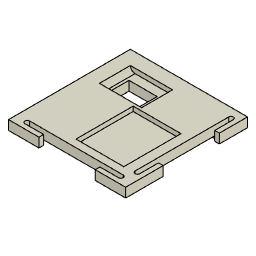
支架2 v23 v1 (Autodesk Fusion 360 design; units mm, degrees)
Autodesk Fusion 360 part; units mm, degrees
sketch "草图1" plane through (0, 0, 0) normal (0, 0, 1) x (1, 0, 0)
  line L0 (57.5, -10) -> (25, -10)
  line L1 (25, -10) -> (25, 0)
  line L2 (25, 0) -> (150, 0)
  line L3 (57.5, -5) -> (57.5, -10)
  line L4 (87.5, 0) -> (117.5, 0)
  arc A0 (137.5, -5) -> (137.5, 0) centre (137.5, -2.5) ccw
  line L5 (150, 30) -> (145, 30)
  arc A1 (37.5, 0) -> (37.5, -5) centre (37.5, -2.5) ccw
  line L6 (150, -10) -> (117.5, -10)
  line L7 (140, 110) -> (140, 60)
  line L8 (150, 120) -> (25, 120)
  line L9 (150, 90) -> (145, 90)
  line L10 (150, 90) -> (150, 120)
  line L11 (87.5, 0) -> (87.5, 120) construction
  line L12 (117.5, -5) -> (117.5, -10)
  line L13 (145, 30) -> (145, 10)
  arc A2 (140, 10) -> (145, 10) centre (142.5, 10) ccw
  line L14 (150, 0) -> (150, 30)
  line L15 (150, 0) -> (150, -10)
  line L16 (137.5, -5) -> (117.5, -5)
  line L17 (140, 10) -> (140, 60)
  line L18 (145, 90) -> (145, 110)
  arc A3 (145, 110) -> (140, 110) centre (142.5, 110) ccw
  line L19 (57.5, -5) -> (37.5, -5)
  line L20 (25, 0) -> (150, 0)
  line L21 (25, 120) -> (25, 0)
  dimension "d1" = 120
  dimension "d2" = 125
  dimension "d3" = 100
  dimension "d4" = 20
  dimension "d5" = 20
  dimension "d6" = 5
  dimension "d7" = 5
  dimension "d8" = 2.5
  dimension "d9" = 2.5
  dimension "d10" = 10
  constraint horizontal L2
  constraint vertical L14
  constraint horizontal L8
  constraint perpendicular L2 L21
  constraint coincident L9.start L14
  constraint perpendicular L9 L14
  constraint perpendicular L9 L18
  constraint tangent L7 A3
  constraint collinear L10 L14
  constraint midpoint L11.end L8
  constraint tangent A0 L16
  constraint tangent A1 L16
  constraint vertical L15
  constraint horizontal L6
  constraint vertical L1
  constraint coincident L0.start L6
  constraint perpendicular L3 L6
  constraint perpendicular L6 L12
  constraint collinear L16 L19
  constraint collinear L0 L6
  constraint coincident A1.start L2
  constraint coincident A0.end L2
  measures "d1" distance of L2 L8
  measures "d2" distance of L14 L21
  measures "d3" distance of A0.start A1.end
  measures "d4" distance of A0.start L12.start
  measures "d5" distance of A1.end L3.start
  measures "d6" distance of L12.start L6.end
  measures "d7" distance of L0.start L3.start
  measures "d8" radius of A0
  measures "d9" radius of A1
  measures "d10" distance of L0 L20
extrude "拉伸1" add sketch "草图1" along normal blind 10 makes body 1
sketch "草图2" plane through (0, 0, 0) normal (0, 0, -1) x (1, 0, 0)
  line L0 (150, -120) -> (150, -90)
  line L1 (150, -90) -> (145, -90)
  line L2 (145, -90) -> (145, -110)
  arc A0 (140, -110) -> (145, -110) centre (142.5, -110) ccw
  line L3 (140, -110) -> (140, -10)
  arc A1 (145, -10) -> (140, -10) centre (142.5, -10) ccw
  line L4 (145, -10) -> (145, -30)
  line L5 (145, -30) -> (150, -30)
  line L6 (150, -30) -> (150, 10)
  line L7 (150, 10) -> (117.5, 10)
  line L8 (117.5, 10) -> (117.5, 5)
  line L9 (117.5, 5) -> (137.5, 5)
  arc A2 (137.5, 0) -> (137.5, 5) centre (137.5, 2.5) ccw
  line L10 (137.5, 0) -> (37.5, 0)
  arc A3 (37.5, 5) -> (37.5, 0) centre (37.5, 2.5) ccw
  line L11 (37.5, 5) -> (57.5, 5)
  line L12 (57.5, 5) -> (57.5, 10)
  line L13 (57.5, 10) -> (25, 10)
  line L14 (25, 10) -> (25, -120)
  line L15 (25, -120) -> (150, -120)
  line L16 (45.5, -10.5) -> (119.5, -10.5)
  line L17 (129.5, -20.5) -> (129.5, -99.5)
  line L18 (119.5, -109.5) -> (45.5, -109.5)
  line L19 (35.5, -99.5) -> (35.5, -20.5)
  arc A4 (45.5, -10.5) -> (35.5, -20.5) centre (45.5, -20.5) ccw
  arc A5 (129.5, -20.5) -> (119.5, -10.5) centre (119.5, -20.5) ccw
  arc A6 (119.5, -109.5) -> (129.5, -99.5) centre (119.5, -99.5) ccw
  arc A7 (35.5, -99.5) -> (45.5, -109.5) centre (45.5, -99.5) ccw
  point P0 (35.5, -10.5)
  point P1 (129.5, -10.5)
  point P2 (35.5, -109.5)
  dimension "d13" = 94
  dimension "d14" = 99
  dimension "d15" = 10.5
  dimension "d16" = 10.5
  dimension "d17" = 10.5
  dimension "d18" = 10.5
  dimension "d19" = 10
  dimension "d20" = 10
  dimension "d21" = 10
  dimension "d22" = 10
  constraint horizontal L16
  constraint vertical L17
  constraint horizontal L18
  constraint vertical L19
  constraint coincident P0 L16
  constraint coincident P0 L19
  constraint tangent L16 A4
  constraint tangent L19 A4
  constraint coincident P1 L16
  constraint coincident P1 L17
  constraint tangent L16 A5
  constraint tangent L17 A5
  constraint tangent L17 A6
  constraint tangent L18 A6
  constraint coincident P2 L19
  constraint coincident P2 L18
  constraint tangent L19 A7
  constraint tangent L18 A7
  measures "d13" distance of P0 P1
  measures "d14" distance of P0 P2
  measures "d15" distance of L3 L17
  measures "d16" distance of L15 L18
  measures "d17" distance of L14 L19
  measures "d18" distance of L10 L16
  measures "d19" radius of A4
  measures "d20" radius of A5
  measures "d21" radius of A6
  measures "d22" radius of A7
extrude "拉伸2" add sketch "草图2" along normal blind 5 contours L16 L17 L18 L19 A4 A5 A6 A7 bodies 1
sketch "草图3" plane through (0, 0, 0) normal (0, 0, -1) x (1, 0, 0)
  line L0 (45.5, -10.5) -> (119.5, -10.5)
  arc A0 (129.5, -20.5) -> (119.5, -10.5) centre (119.5, -20.5) ccw
  line L1 (129.5, -20.5) -> (129.5, -99.5)
  arc A1 (119.5, -109.5) -> (129.5, -99.5) centre (119.5, -99.5) ccw
  line L2 (119.5, -109.5) -> (45.5, -109.5)
  arc A2 (35.5, -99.5) -> (45.5, -109.5) centre (45.5, -99.5) ccw
  line L3 (35.5, -99.5) -> (35.5, -20.5)
  arc A3 (45.5, -10.5) -> (35.5, -20.5) centre (45.5, -20.5) ccw
  line L4 (150, -120) -> (150, -90)
  line L5 (150, -90) -> (145, -90)
  line L6 (145, -90) -> (145, -110)
  arc A4 (140, -110) -> (145, -110) centre (142.5, -110) ccw
  line L7 (140, -110) -> (140, -10)
  arc A5 (145, -10) -> (140, -10) centre (142.5, -10) ccw
  line L8 (145, -10) -> (145, -30)
  line L9 (145, -30) -> (150, -30)
  line L10 (150, -30) -> (150, 10)
  line L11 (150, 10) -> (117.5, 10)
  line L12 (117.5, 10) -> (117.5, 5)
  line L13 (117.5, 5) -> (137.5, 5)
  arc A6 (137.5, 0) -> (137.5, 5) centre (137.5, 2.5) ccw
  line L14 (137.5, 0) -> (37.5, 0)
  arc A7 (37.5, 5) -> (37.5, 0) centre (37.5, 2.5) ccw
  line L15 (37.5, 5) -> (57.5, 5)
  line L16 (57.5, 5) -> (57.5, 10)
  line L17 (57.5, 10) -> (25, 10)
  line L18 (25, 10) -> (25, -120)
  line L19 (25, -120) -> (150, -120)
  line L20 (30.5, -5.5) -> (44.5, -5.5)
  line L21 (44.5, -5.5) -> (44.5, -7.5)
  line L22 (44.5, -7.5) -> (32.5, -7.5)
  line L23 (30.5, -7.5) -> (30.5, -5.5)
  line L24 (30.5, -5.5) -> (33.5, -5.5)
  line L25 (32.5, -7.5) -> (32.5, -19.5)
  line L26 (32.5, -19.5) -> (30.5, -19.5)
  line L27 (30.5, -19.5) -> (30.5, -5.5)
  line L28 (120.5, -5.5) -> (134.5, -5.5)
  line L29 (134.5, -5.5) -> (134.5, -8.5)
  line L30 (132.5, -7.5) -> (120.5, -7.5)
  line L31 (120.5, -7.5) -> (120.5, -5.5)
  line L32 (134.5, -5.5) -> (131.5, -5.5)
  line L33 (132.5, -7.5) -> (132.5, -19.5)
  line L34 (132.5, -19.5) -> (134.5, -19.5)
  line L35 (134.5, -19.5) -> (134.5, -5.5)
  line L36 (30.5, -100.5) -> (32.5, -100.5)
  line L37 (32.5, -100.5) -> (32.5, -112.5)
  line L38 (33.5, -114.5) -> (30.5, -114.5)
  line L39 (30.5, -114.5) -> (30.5, -100.5)
  line L40 (30.5, -114.5) -> (44.5, -114.5)
  line L41 (44.5, -114.5) -> (44.5, -112.5)
  line L42 (44.5, -112.5) -> (32.5, -112.5)
  line L43 (30.5, -111.5) -> (30.5, -114.5)
  line L44 (120.5, -112.5) -> (132.5, -112.5)
  line L45 (134.5, -112.5) -> (134.5, -114.5)
  line L46 (134.5, -114.5) -> (120.5, -114.5)
  line L47 (120.5, -114.5) -> (120.5, -112.5)
  line L48 (134.5, -114.5) -> (131.5, -114.5)
  line L49 (132.5, -112.5) -> (132.5, -100.5)
  line L50 (132.5, -100.5) -> (134.5, -100.5)
  line L51 (134.5, -100.5) -> (134.5, -114.5)
  dimension "d28" = 14
  dimension "d29" = 5.5
  dimension "d30" = 5.5
  dimension "d31" = 14
  dimension "d32" = 2
  dimension "d34" = 14
  dimension "d35" = 5.5
  dimension "d36" = 5.5
  dimension "d37" = 2
  dimension "d38" = 14
  dimension "d39" = 14
  dimension "d41" = 5.5
  dimension "d42" = 5.5
  dimension "d43" = 14
  dimension "d44" = 2
  dimension "d45" = 14
  dimension "d46" = 5.5
  dimension "d47" = 5.5
  dimension "d107" = 2
  dimension "d108" = 14
  dimension "d109" = 2
  dimension "d110" = 2
  dimension "d111" = 2
  dimension "d112" = 2
  constraint horizontal L20
  constraint vertical L21
  constraint horizontal L22
  constraint vertical L23
  constraint horizontal L24
  constraint vertical L25
  constraint horizontal L26
  constraint vertical L27
  constraint horizontal L28
  constraint vertical L29
  constraint horizontal L30
  constraint vertical L31
  constraint horizontal L32
  constraint vertical L33
  constraint horizontal L34
  constraint vertical L35
  constraint horizontal L36
  constraint vertical L37
  constraint horizontal L38
  constraint vertical L39
  constraint horizontal L40
  constraint vertical L41
  constraint horizontal L42
  constraint vertical L43
  constraint horizontal L44
  constraint vertical L45
  constraint horizontal L46
  constraint vertical L47
  constraint horizontal L48
  constraint vertical L49
  constraint horizontal L50
  constraint vertical L51
  measures "d28" distance of L20.start L26.end
  measures "d29" distance of L14 L20
  measures "d30" distance of L18 L27
  measures "d31" distance of L28.start L28.end
  measures "d32" distance of L28.start L30.end
  measures "d34" distance of L28.end L34.end
  measures "d35" distance of L7 L35
  measures "d36" distance of L14 L28
  measures "d37" distance of L36.start L36.end
  measures "d38" distance of L36.start L38.end
  measures "d39" distance of L38.end L40.end
  measures "d41" distance of L19 L40
  measures "d42" distance of L18 L39
  measures "d43" distance of L44.start L45.start
  measures "d44" distance of L44.start L46.end
  measures "d45" distance of L45.end L50.end
  measures "d46" distance of L19 L46
  measures "d47" distance of L7 L51
  measures "d107" distance of L20.end L21.end
  measures "d108" distance of L20.start L20.end
  measures "d109" distance of L25.end L26.end
  measures "d110" distance of L33.end L34.end
  measures "d111" distance of L49.end L50.end
  measures "d112" distance of L40.end L41.end
extrude "拉伸3" add sketch "草图3" along normal blind 8 contours L20 L21 L22 L23 L24 L25 L26 L27 | L28 L29 L30 L31 L32 L33 L34 L35 | L36 L37 L38 L39 L40 L41 L42 L43 | L44 L45 L46 L47 L48 L49 L50 L51 bodies 1
sketch "草图4" plane through (0, 0, 10) normal (0, 0, 1) x (-1, 0, 0)
  line L0 (-150, -90) -> (-150, -120)
  line L1 (-150, -120) -> (-25, -120)
  line L2 (-25, -120) -> (-25, 10)
  line L3 (-25, 10) -> (-57.5, 10)
  line L4 (-57.5, 10) -> (-57.5, 5)
  line L5 (-57.5, 5) -> (-37.5, 5)
  arc A0 (-37.5, 0) -> (-37.5, 5) centre (-37.5, 2.5) ccw
  line L6 (-37.5, 0) -> (-137.5, 0)
  arc A1 (-137.5, 5) -> (-137.5, 0) centre (-137.5, 2.5) ccw
  line L7 (-137.5, 5) -> (-117.5, 5)
  line L8 (-117.5, 5) -> (-117.5, 10)
  line L9 (-117.5, 10) -> (-150, 10)
  line L10 (-150, 10) -> (-150, -30)
  line L11 (-150, -30) -> (-145, -30)
  line L12 (-145, -30) -> (-145, -10)
  arc A2 (-140, -10) -> (-145, -10) centre (-142.5, -10) ccw
  line L13 (-140, -10) -> (-140, -110)
  arc A3 (-145, -110) -> (-140, -110) centre (-142.5, -110) ccw
  line L14 (-145, -110) -> (-145, -90)
  line L15 (-145, -90) -> (-150, -90)
  line L16 (-40, -105) -> (-85, -105)
  line L17 (-85, -105) -> (-85, -72)
  line L18 (-85, -72) -> (-40, -72)
  line L19 (-40, -72) -> (-40, -105)
  dimension "d50" = 45
  dimension "d51" = 33
  dimension "d52" = 15
  dimension "d53" = 15
  constraint horizontal L16
  constraint vertical L17
  constraint horizontal L18
  constraint vertical L19
  measures "d50" distance of L16.start L16.end
  measures "d51" distance of L16.start L18.end
  measures "d52" distance of L1 L16
  measures "d53" distance of L2 L19
extrude "拉伸4" cut sketch "草图4" against normal blind 5 contours L16 L17 L18 L19 bodies 1
fillet "圆角1" radius 5 1 edges at (40, 88.5, 5) on bodies 1
fillet "圆角2" radius 5 1 edges at (85, 88.5, 5) on bodies 1
sketch "草图5" plane through (0, 0, 10) normal (0, 0, 1) x (-1, 0, 0)
  line L0 (-85, -105) -> (-85, -72)
  line L1 (-85, -72) -> (-40, -72)
  line L2 (-40, -72) -> (-40, -105)
  line L3 (-40, -105) -> (-85, -105)
  line L4 (-150, -90) -> (-150, -120)
  line L5 (-150, -120) -> (-25, -120)
  line L6 (-25, -120) -> (-25, 10)
  line L7 (-25, 10) -> (-57.5, 10)
  line L8 (-57.5, 10) -> (-57.5, 5)
  line L9 (-57.5, 5) -> (-37.5, 5)
  arc A0 (-37.5, 0) -> (-37.5, 5) centre (-37.5, 2.5) ccw
  line L10 (-37.5, 0) -> (-137.5, 0)
  arc A1 (-137.5, 5) -> (-137.5, 0) centre (-137.5, 2.5) ccw
  line L11 (-137.5, 5) -> (-117.5, 5)
  line L12 (-117.5, 5) -> (-117.5, 10)
  line L13 (-117.5, 10) -> (-150, 10)
  line L14 (-150, 10) -> (-150, -30)
  line L15 (-150, -30) -> (-145, -30)
  line L16 (-145, -30) -> (-145, -10)
  arc A2 (-140, -10) -> (-145, -10) centre (-142.5, -10) ccw
  line L17 (-140, -10) -> (-140, -110)
  arc A3 (-145, -110) -> (-140, -110) centre (-142.5, -110) ccw
  line L18 (-145, -110) -> (-145, -90)
  line L19 (-145, -90) -> (-150, -90)
  line L20 (-79, -69) -> (-130, -69)
  line L21 (-130, -69) -> (-130, -8)
  line L22 (-130, -8) -> (-79, -8)
  line L23 (-79, -8) -> (-79, -69)
  dimension "d60" = 10
  dimension "d61" = 8
  dimension "d113" = 61
  dimension "d114" = 51
  constraint horizontal L20
  constraint vertical L21
  constraint horizontal L22
  constraint vertical L23
  measures "d60" distance of L17 L21
  measures "d61" distance of L10 L22
  measures "d113" distance of L20.start L22.end
  measures "d114" distance of L20.start L20.end
sketch "草图12" plane through (0, 0, 5) normal (0, 0, 1) x (-1, 0, 0)
  line L0 (-80, -72) -> (-80, -105)
  line L1 (-80, -105) -> (-45, -105)
  line L2 (-45, -105) -> (-45, -72)
  line L3 (-45, -72) -> (-80, -72)
  line L4 (-85, -72) -> (-40, -72)
  line L5 (-48, -95.6) -> (-78, -95.6)
  line L6 (-78, -95.6) -> (-78, -77)
  line L7 (-78, -77) -> (-48, -77)
  line L8 (-48, -77) -> (-48, -95.6)
  dimension "d92" = 30
  dimension "d93" = 18.6
  dimension "d94" = 5
  dimension "d95" = 2
  constraint horizontal L5
  constraint vertical L6
  constraint horizontal L7
  constraint vertical L8
  measures "d92" distance of L5.start L5.end
  measures "d93" distance of L5.start L7.end
  measures "d94" distance of L4 L7
  measures "d95" distance of L0 L6
extrude "拉伸13" cut sketch "草图12" against normal blind 11 contours L5 L6 L7 L8 bodies 1
copy_body "实体->零部件2" bodies 1 removing the originals makes body 2 in component "支架2"
extrude "拉伸1'" cut sketch "草图5" against normal blind 5 contours L20 L21 L22 L23 bodies 2 in component "支架2"
component "支架2" placed x (1, 0, 0) y (0, 1, 0) z (0, 0, 1) at (0, 0, 0)
